Autodesk Fusion 360 part; units mm, degrees
(part 5 of 8)
  spline S142 degree 5 poles (498.6725, -294.9889) (498.7009, -294.8971) (498.7576, -294.7134) (498.842, -294.4377) (498.9535, -294.0701) (499.0912, -293.6105) (499.227, -293.1507) (499.3612, -292.6907) (499.4936, -292.2306) (499.6242, -291.7704) (499.753, -291.31) (499.88, -290.8494) (500.0052, -290.3888) (500.1286, -289.928) (500.2501, -289.4671) (500.3698, -289.006) (500.4876, -288.5449) (500.6035, -288.0836) (500.7175, -287.6223) (500.8296, -287.1608) (500.9398, -286.6992) (501.048, -286.2376) (501.1543, -285.7758) (501.2586, -285.314) (501.3609, -284.8521) (501.4612, -284.3901) (501.5595, -283.9281) (501.6557, -283.4659) (501.7499, -283.0038) (501.842, -282.5415) (501.9319, -282.0793) (502.0198, -281.617) (502.1054, -281.1546) (502.1889, -280.6922) (502.2703, -280.2298) (502.3493, -279.7674) (502.4262, -279.305) (502.5007, -278.8425) (502.5729, -278.3801) (502.6428, -277.9177) (502.7103, -277.4553) (502.7755, -276.9929) (502.8382, -276.5306) (502.8984, -276.0683) (502.9562, -275.606) (503.0114, -275.1439) (503.0639, -274.6817) (503.1139, -274.2197) (503.1611, -273.7578) (503.2055, -273.2959) (503.2472, -272.8342) (503.2861, -272.3726) (503.3222, -271.9111) (503.3553, -271.4498) (503.3854, -270.9886) (503.4124, -270.5277) (503.436, -270.0669) (503.4562, -269.6064) (503.4729, -269.1461) (503.4861, -268.6861) (503.4957, -268.2264) (503.501, -267.8309) (503.5031, -267.5274) (503.5035, -267.3158) (503.5034, -267.1961) (503.5034, -267.1682) knots -1 -1 -1 -1 -1 -1 -0.98571429 -0.97142857 -0.95714286 -0.94285714 -0.92857143 -0.91428571 -0.9 -0.88571429 -0.87142857 -0.85714286 -0.84285714 -0.82857143 -0.81428571 -0.8 -0.78571429 -0.77142857 -0.75714286 -0.74285714 -0.72857143 -0.71428571 -0.7 -0.68571429 -0.67142857 -0.65714286 -0.64285714 -0.62857143 -0.61428571 -0.6 -0.58571429 -0.57142857 -0.55714286 -0.54285714 -0.52857143 -0.51428571 -0.5 -0.48571429 -0.47142857 -0.45714286 -0.44285714 -0.42857143 -0.41428571 -0.4 -0.38571429 -0.37142857 -0.35714286 -0.34285714 -0.32857143 -0.31428571 -0.3 -0.28571429 -0.27142857 -0.25714286 -0.24285714 -0.22857143 -0.21428571 -0.2 -0.18571429 -0.17142857 -0.15714286 -0.14285714 -0.13851185 -0.13851185 -0.13851185 -0.13851185 -0.13851185 -0.13851185
  spline S143 degree 3 poles (504.8034, -265.6048) (504.6001, -265.6422) (504.406, -265.719) (504.0583, -265.9427) (503.908, -266.0874) (503.6968, -266.3896) (503.6248, -266.5359) (503.5278, -266.8451) (503.5032, -267.0062) (503.5034, -267.1682) knots 0 0 0 0 0.062015 0.062015 0.12403 0.12403 0.172638 0.172638 0.221247 0.221247 0.221247 0.221247
  arc A72 (504.8034, -265.6048) -> (512.8852, -263.9972) centre (452.3696, 19.1166) ccw
  spline S144 degree 3 poles (514.6845, -264.9442) (514.6056, -264.7531) (514.4902, -264.5792) (514.1992, -264.2855) (514.0265, -264.1685) (513.6869, -264.0247) (513.5289, -263.9847) (513.2063, -263.954) (513.0436, -263.9634) (512.8852, -263.9972) knots 0 0 0 0 0.062015 0.062015 0.12403 0.12403 0.172638 0.172638 0.221247 0.221247 0.221247 0.221247
  spline S145 degree 5 poles (514.6845, -264.9442) (514.6951, -264.97) (514.7409, -265.0806) (514.8222, -265.2759) (514.9403, -265.5554) (515.0965, -265.9188) (515.2814, -266.3399) (515.4696, -266.7598) (515.6611, -267.1787) (515.856, -267.5964) (516.0542, -268.013) (516.2555, -268.4286) (516.4598, -268.8432) (516.6669, -269.2567) (516.8768, -269.6693) (517.0894, -270.0808) (517.3047, -270.4915) (517.5225, -270.9011) (517.7429, -271.3098) (517.9658, -271.7176) (518.1912, -272.1244) (518.4191, -272.5303) (518.6493, -272.9353) (518.8819, -273.3393) (519.1168, -273.7425) (519.3539, -274.1447) (519.5932, -274.5461) (519.8347, -274.9465) (520.0784, -275.3461) (520.3243, -275.7448) (520.5722, -276.1427) (520.8222, -276.5396) (521.0743, -276.9357) (521.3284, -277.3309) (521.5845, -277.7253) (521.8426, -278.1188) (522.1026, -278.5115) (522.3645, -278.9033) (522.6284, -279.2942) (522.8941, -279.6843) (523.1617, -280.0736) (523.4312, -280.4621) (523.7025, -280.8496) (523.9756, -281.2364) (524.2505, -281.6223) (524.5272, -282.0074) (524.8056, -282.3917) (525.0858, -282.7751) (525.3677, -283.1577) (525.6513, -283.5395) (525.9366, -283.9205) (526.2236, -284.3006) (526.5122, -284.68) (526.8025, -285.0585) (527.0945, -285.4361) (527.3881, -285.813) (527.6833, -286.1891) (527.9801, -286.5643) (528.2784, -286.9387) (528.5784, -287.3123) (528.8799, -287.6851) (529.183, -288.0571) (529.4267, -288.3541) (529.6101, -288.5764) (529.7328, -288.7245) (529.7942, -288.7985) knots 0.13851185 0.13851185 0.13851185 0.13851185 0.13851185 0.13851185 0.14285714 0.15714286 0.17142857 0.18571429 0.2 0.21428571 0.22857143 0.24285714 0.25714286 0.27142857 0.28571429 0.3 0.31428571 0.32857143 0.34285714 0.35714286 0.37142857 0.38571429 0.4 0.41428571 0.42857143 0.44285714 0.45714286 0.47142857 0.48571429 0.5 0.51428571 0.52857143 0.54285714 0.55714286 0.57142857 0.58571429 0.6 0.61428571 0.62857143 0.64285714 0.65714286 0.67142857 0.68571429 0.7 0.71428571 0.72857143 0.74285714 0.75714286 0.77142857 0.78571429 0.8 0.81428571 0.82857143 0.84285714 0.85714286 0.87142857 0.88571429 0.9 0.91428571 0.92857143 0.94285714 0.95714286 0.97142857 0.98571429 1 1 1 1 1 1
  arc A73 (529.7942, -288.7985) -> (539.2754, -286.258) centre (452.3696, 19.1166) ccw
  spline S146 degree 5 poles (539.2754, -286.258) (539.2916, -286.1632) (539.3237, -285.9737) (539.3715, -285.6894) (539.434, -285.3104) (539.5105, -284.8367) (539.5852, -284.3631) (539.6582, -283.8895) (539.7294, -283.4161) (539.7988, -282.9427) (539.8664, -282.4695) (539.9322, -281.9963) (539.9962, -281.5232) (540.0584, -281.0503) (540.1187, -280.5774) (540.1772, -280.1047) (540.2338, -279.6322) (540.2885, -279.1597) (540.3413, -278.6874) (540.3923, -278.2153) (540.4412, -277.7433) (540.4883, -277.2714) (540.5334, -276.7998) (540.5765, -276.3283) (540.6177, -275.8569) (540.6568, -275.3858) (540.694, -274.9149) (540.729, -274.4442) (540.7621, -273.9737) (540.793, -273.5034) (540.8219, -273.0333) (540.8486, -272.5635) (540.8732, -272.0939) (540.8956, -271.6246) (540.9159, -271.1555) (540.9339, -270.6867) (540.9497, -270.2182) (540.9633, -269.75) (540.9745, -269.2821) (540.9835, -268.8146) (540.9901, -268.3473) (540.9943, -267.8804) (540.9961, -267.4138) (540.9955, -266.9476) (540.9924, -266.4818) (540.9868, -266.0163) (540.9786, -265.5513) (540.9678, -265.0867) (540.9543, -264.6226) (540.9381, -264.1589) (540.9192, -263.6957) (540.8975, -263.2329) (540.873, -262.7707) (540.8457, -262.309) (540.8153, -261.8478) (540.7819, -261.3873) (540.7452, -260.9274) (540.7051, -260.4682) (540.6615, -260.0097) (540.6146, -259.5519) (540.5641, -259.0948) (540.5177, -258.702) (540.4802, -258.4008) (540.453, -258.191) (540.4373, -258.0724) (540.4336, -258.0447) knots -1 -1 -1 -1 -1 -1 -0.98571429 -0.97142857 -0.95714286 -0.94285714 -0.92857143 -0.91428571 -0.9 -0.88571429 -0.87142857 -0.85714286 -0.84285714 -0.82857143 -0.81428571 -0.8 -0.78571429 -0.77142857 -0.75714286 -0.74285714 -0.72857143 -0.71428571 -0.7 -0.68571429 -0.67142857 -0.65714286 -0.64285714 -0.62857143 -0.61428571 -0.6 -0.58571429 -0.57142857 -0.55714286 -0.54285714 -0.52857143 -0.51428571 -0.5 -0.48571429 -0.47142857 -0.45714286 -0.44285714 -0.42857143 -0.41428571 -0.4 -0.38571429 -0.37142857 -0.35714286 -0.34285714 -0.32857143 -0.31428571 -0.3 -0.28571429 -0.27142857 -0.25714286 -0.24285714 -0.22857143 -0.21428571 -0.2 -0.18571429 -0.17142857 -0.15714286 -0.14285714 -0.13851185 -0.13851185 -0.13851185 -0.13851185 -0.13851185 -0.13851185
  spline S147 degree 3 poles (541.5184, -256.325) (541.3217, -256.3886) (541.1394, -256.4901) (540.8238, -256.7572) (540.6936, -256.9203) (540.5237, -257.2476) (540.4715, -257.4019) (540.4156, -257.7211) (540.4122, -257.8841) (540.4336, -258.0447) knots 0 0 0 0 0.062015 0.062015 0.12403 0.12403 0.172638 0.172638 0.221247 0.221247 0.221247 0.221247
  arc A74 (541.5184, -256.325) -> (549.3212, -253.6763) centre (452.3696, 19.1166) ccw
  spline S148 degree 3 poles (551.2287, -254.3803) (551.1256, -254.2011) (550.9885, -254.0438) (550.6617, -253.7906) (550.4751, -253.6971) (550.1197, -253.5988) (549.9578, -253.5798) (549.634, -253.5915) (549.4739, -253.622) (549.3212, -253.6763) knots 0 0 0 0 0.062015 0.062015 0.12403 0.12403 0.172638 0.172638 0.221247 0.221247 0.221247 0.221247
  spline S149 degree 5 poles (551.2287, -254.3803) (551.2427, -254.4044) (551.3024, -254.5082) (551.4086, -254.6911) (551.5621, -254.9529) (551.7645, -255.2928) (552.0027, -255.6861) (552.2441, -256.0779) (552.4887, -256.4682) (552.7364, -256.8569) (552.9873, -257.2441) (553.2411, -257.6298) (553.4978, -258.0142) (553.7571, -258.3971) (554.0191, -258.7788) (554.2836, -259.1591) (554.5506, -259.5381) (554.82, -259.9158) (555.0918, -260.2923) (555.3661, -260.6674) (555.6427, -261.0413) (555.9216, -261.414) (556.2027, -261.7855) (556.486, -262.1557) (556.7715, -262.5247) (557.0591, -262.8926) (557.3488, -263.2593) (557.6405, -263.6248) (557.9343, -263.9892) (558.23, -264.3524) (558.5278, -264.7144) (558.8275, -265.0754) (559.1291, -265.4352) (559.4326, -265.7938) (559.738, -266.1514) (560.0452, -266.5079) (560.3543, -266.8632) (560.6651, -267.2175) (560.9777, -267.5707) (561.2921, -267.9228) (561.6083, -268.2738) (561.9261, -268.6237) (562.2457, -268.9726) (562.5669, -269.3204) (562.8898, -269.6671) (563.2144, -270.0128) (563.5406, -270.3574) (563.8684, -270.701) (564.1979, -271.0436) (564.5289, -271.3851) (564.8615, -271.7255) (565.1956, -272.065) (565.5313, -272.4034) (565.8686, -272.7407) (566.2073, -273.0771) (566.5476, -273.4124) (566.8893, -273.7467) (567.2326, -274.08) (567.5773, -274.4123) (567.9234, -274.7435) (568.271, -275.0738) (568.62, -275.403) (568.9004, -275.6656) (569.1113, -275.8621) (569.2522, -275.9929) (569.3228, -276.0583) knots 0.13851185 0.13851185 0.13851185 0.13851185 0.13851185 0.13851185 0.14285714 0.15714286 0.17142857 0.18571429 0.2 0.21428571 0.22857143 0.24285714 0.25714286 0.27142857 0.28571429 0.3 0.31428571 0.32857143 0.34285714 0.35714286 0.37142857 0.38571429 0.4 0.41428571 0.42857143 0.44285714 0.45714286 0.47142857 0.48571429 0.5 0.51428571 0.52857143 0.54285714 0.55714286 0.57142857 0.58571429 0.6 0.61428571 0.62857143 0.64285714 0.65714286 0.67142857 0.68571429 0.7 0.71428571 0.72857143 0.74285714 0.75714286 0.77142857 0.78571429 0.8 0.81428571 0.82857143 0.84285714 0.85714286 0.87142857 0.88571429 0.9 0.91428571 0.92857143 0.94285714 0.95714286 0.97142857 0.98571429 1 1 1 1 1 1
  arc A75 (569.3228, -276.0583) -> (578.3913, -272.302) centre (452.3696, 19.1166) ccw
  spline S150 degree 5 poles (578.3913, -272.302) (578.395, -272.2059) (578.4021, -272.0138) (578.4123, -271.7257) (578.4249, -271.3417) (578.4389, -270.8621) (578.4511, -270.3828) (578.4617, -269.9038) (578.4704, -269.4251) (578.4775, -268.9468) (578.4827, -268.4687) (578.4862, -267.991) (578.4879, -267.5136) (578.4878, -267.0366) (578.4859, -266.5599) (578.4822, -266.0837) (578.4766, -265.6077) (578.4692, -265.1322) (578.4599, -264.657) (578.4488, -264.1823) (578.4358, -263.7079) (578.4208, -263.234) (578.404, -262.7605) (578.3852, -262.2874) (578.3645, -261.8147) (578.3418, -261.3425) (578.3171, -260.8708) (578.2905, -260.3995) (578.2618, -259.9287) (578.2311, -259.4584) (578.1984, -258.9886) (578.1635, -258.5193) (578.1266, -258.0505) (578.0876, -257.5823) (578.0465, -257.1146) (578.0032, -256.6475) (577.9577, -256.1809) (577.91, -255.7149) (577.8601, -255.2496) (577.8079, -254.7848) (577.7535, -254.3207) (577.6967, -253.8572) (577.6376, -253.3944) (577.5762, -252.9323) (577.5123, -252.4708) (577.446, -252.0101) (577.3772, -251.5501) (577.3058, -251.0909) (577.2319, -250.6325) (577.1553, -250.1749) (577.0761, -249.7181) (576.9942, -249.2622) (576.9096, -248.8071) (576.8222, -248.3529) (576.7319, -247.8997) (576.6386, -247.4474) (576.5422, -246.9962) (576.4425, -246.5462) (576.3395, -246.0973) (576.2331, -245.6495) (576.1235, -245.203) (576.0262, -244.8196) (575.9497, -244.5259) (575.8953, -244.3214) (575.8643, -244.2058) (575.857, -244.1789) knots -1 -1 -1 -1 -1 -1 -0.98571429 -0.97142857 -0.95714286 -0.94285714 -0.92857143 -0.91428571 -0.9 -0.88571429 -0.87142857 -0.85714286 -0.84285714 -0.82857143 -0.81428571 -0.8 -0.78571429 -0.77142857 -0.75714286 -0.74285714 -0.72857143 -0.71428571 -0.7 -0.68571429 -0.67142857 -0.65714286 -0.64285714 -0.62857143 -0.61428571 -0.6 -0.58571429 -0.57142857 -0.55714286 -0.54285714 -0.52857143 -0.51428571 -0.5 -0.48571429 -0.47142857 -0.45714286 -0.44285714 -0.42857143 -0.41428571 -0.4 -0.38571429 -0.37142857 -0.35714286 -0.34285714 -0.32857143 -0.31428571 -0.3 -0.28571429 -0.27142857 -0.25714286 -0.24285714 -0.22857143 -0.21428571 -0.2 -0.18571429 -0.17142857 -0.15714286 -0.14285714 -0.13851185 -0.13851185 -0.13851185 -0.13851185 -0.13851185 -0.13851185
  spline S151 degree 3 poles (576.7081, -242.3323) (576.5214, -242.4211) (576.3538, -242.5455) (576.0758, -242.8515) (575.9681, -243.0302) (575.8423, -243.3768) (575.8107, -243.5367) (575.7969, -243.8604) (575.8149, -244.0224) (575.857, -244.1789) knots 0 0 0 0 0.062015 0.062015 0.12403 0.12403 0.172638 0.172638 0.221247 0.221247 0.221247 0.221247
  arc A76 (576.7081, -242.3323) -> (584.0984, -238.6878) centre (452.3696, 19.1166) ccw
  spline S152 degree 3 poles (586.0815, -239.1367) (585.9559, -238.9726) (585.7994, -238.8345) (585.4423, -238.6261) (585.2451, -238.5578) (584.8799, -238.5068) (584.717, -238.5091) (584.3974, -238.5628) (584.2427, -238.6141) (584.0984, -238.6878) knots 0 0 0 0 0.062015 0.062015 0.12403 0.12403 0.172638 0.172638 0.221247 0.221247 0.221247 0.221247
  spline S153 degree 5 poles (586.0815, -239.1367) (586.0984, -239.1589) (586.1713, -239.2539) (586.3004, -239.4215) (586.4868, -239.661) (586.7317, -239.9716) (587.0193, -240.3304) (587.3097, -240.6873) (587.6032, -241.0423) (587.8996, -241.3954) (588.1988, -241.7465) (588.5008, -242.0959) (588.8054, -242.4434) (589.1125, -242.7892) (589.4221, -243.1334) (589.734, -243.4759) (590.0481, -243.8169) (590.3646, -244.1562) (590.6832, -244.4939) (591.0041, -244.8301) (591.3271, -245.1647) (591.6523, -245.4978) (591.9795, -245.8294) (592.3087, -246.1595) (592.6399, -246.4881) (592.973, -246.8153) (593.3081, -247.141) (593.6451, -247.4653) (593.9839, -247.7882) (594.3245, -248.1097) (594.667, -248.4298) (595.0112, -248.7485) (595.3572, -249.0659) (595.7049, -249.3819) (596.0544, -249.6965) (596.4055, -250.0098) (596.7583, -250.3218) (597.1127, -250.6325) (597.4688, -250.9418) (597.8264, -251.2498) (598.1857, -251.5566) (598.5465, -251.8621) (598.9088, -252.1662) (599.2727, -252.4691) (599.6382, -252.7707) (600.0051, -253.0711) (600.3735, -253.3702) (600.7433, -253.6681) (601.1147, -253.9647) (601.4874, -254.2601) (601.8616, -254.5542) (602.2372, -254.8471) (602.6142, -255.1388) (602.9926, -255.4293) (603.3723, -255.7185) (603.7535, -256.0066) (604.1359, -256.2934) (604.5197, -256.579) (604.9048, -256.8635) (605.2913, -257.1467) (605.679, -257.4288) (606.068, -257.7097) (606.3803, -257.9334) (606.615, -258.1007) (606.7718, -258.212) (606.8503, -258.2676) knots 0.13851185 0.13851185 0.13851185 0.13851185 0.13851185 0.13851185 0.14285714 0.15714286 0.17142857 0.18571429 0.2 0.21428571 0.22857143 0.24285714 0.25714286 0.27142857 0.28571429 0.3 0.31428571 0.32857143 0.34285714 0.35714286 0.37142857 0.38571429 0.4 0.41428571 0.42857143 0.44285714 0.45714286 0.47142857 0.48571429 0.5 0.51428571 0.52857143 0.54285714 0.55714286 0.57142857 0.58571429 0.6 0.61428571 0.62857143 0.64285714 0.65714286 0.67142857 0.68571429 0.7 0.71428571 0.72857143 0.74285714 0.75714286 0.77142857 0.78571429 0.8 0.81428571 0.82857143 0.84285714 0.85714286 0.87142857 0.88571429 0.9 0.91428571 0.92857143 0.94285714 0.95714286 0.97142857 0.98571429 1 1 1 1 1 1
  arc A77 (606.8503, -258.2676) -> (615.3509, -253.3597) centre (452.3696, 19.1166) ccw
  spline S154 degree 5 poles (615.3509, -253.3597) (615.342, -253.264) (615.324, -253.0726) (615.2965, -252.7856) (615.2589, -252.4033) (615.2101, -251.926) (615.1597, -251.4492) (615.1077, -250.9729) (615.0539, -250.4971) (614.9984, -250.0219) (614.9412, -249.5473) (614.8823, -249.0732) (614.8217, -248.5997) (614.7594, -248.1268) (614.6953, -247.6545) (614.6294, -247.1827) (614.5618, -246.7116) (614.4923, -246.2411) (614.4211, -245.7712) (614.3481, -245.302) (614.2733, -244.8334) (614.1966, -244.3654) (614.1181, -243.8982) (614.0377, -243.4316) (613.9555, -242.9657) (613.8713, -242.5005) (613.7853, -242.036) (613.6974, -241.5722) (613.6075, -241.1092) (613.5157, -240.6469) (613.4219, -240.1854) (613.3261, -239.7247) (613.2283, -239.2647) (613.1285, -238.8056) (613.0267, -238.3473) (612.9228, -237.8898) (612.8168, -237.4332) (612.7087, -236.9774) (612.5985, -236.5225) (612.4861, -236.0686) (612.3715, -235.6155) (612.2548, -235.1634) (612.1358, -234.7123) (612.0145, -234.2621) (611.891, -233.813) (611.7651, -233.3648) (611.6368, -232.9178) (611.5061, -232.4718) (611.373, -232.027) (611.2373, -231.5833) (611.0991, -231.1407) (610.9584, -230.6994) (610.8152, -230.2592) (610.6692, -229.8203) (610.5206, -229.3828) (610.369, -228.9466) (610.2145, -228.5118) (610.057, -228.0786) (609.8963, -227.647) (609.7324, -227.217) (609.5654, -226.7886) (609.4189, -226.4211) (609.3047, -226.14) (609.2241, -225.9443) (609.1782, -225.8338) (609.1675, -225.808) knots -1 -1 -1 -1 -1 -1 -0.98571429 -0.97142857 -0.95714286 -0.94285714 -0.92857143 -0.91428571 -0.9 -0.88571429 -0.87142857 -0.85714286 -0.84285714 -0.82857143 -0.81428571 -0.8 -0.78571429 -0.77142857 -0.75714286 -0.74285714 -0.72857143 -0.71428571 -0.7 -0.68571429 -0.67142857 -0.65714286 -0.64285714 -0.62857143 -0.61428571 -0.6 -0.58571429 -0.57142857 -0.55714286 -0.54285714 -0.52857143 -0.51428571 -0.5 -0.48571429 -0.47142857 -0.45714286 -0.44285714 -0.42857143 -0.41428571 -0.4 -0.38571429 -0.37142857 -0.35714286 -0.34285714 -0.32857143 -0.31428571 -0.3 -0.28571429 -0.27142857 -0.25714286 -0.24285714 -0.22857143 -0.21428571 -0.2 -0.18571429 -0.17142857 -0.15714286 -0.14285714 -0.13851185 -0.13851185 -0.13851185 -0.13851185 -0.13851185 -0.13851185
  spline S155 degree 3 poles (609.7703, -223.8661) (609.5968, -223.9785) (609.4469, -224.1237) (609.2112, -224.4634) (609.1277, -224.6546) (609.0482, -225.0147) (609.0377, -225.1773) (609.0664, -225.5001) (609.1053, -225.6584) (609.1675, -225.808) knots 0 0 0 0 0.062015 0.062015 0.12403 0.12403 0.172638 0.172638 0.221247 0.221247 0.221247 0.221247
  arc A78 (609.7703, -223.8661) -> (616.6217, -219.2882) centre (452.3696, 19.1166) ccw
  spline S156 degree 3 poles (618.6464, -219.4744) (618.5004, -219.3281) (618.3272, -219.2116) (617.946, -219.0516) (617.7416, -219.0096) (617.3729, -219.0067) (617.2116, -219.0302) (616.9018, -219.1253) (616.7551, -219.1962) (616.6217, -219.2882) knots 0 0 0 0 0.062015 0.062015 0.12403 0.12403 0.172638 0.172638 0.221247 0.221247 0.221247 0.221247
  spline S157 degree 5 poles (618.6464, -219.4744) (618.6661, -219.4942) (618.7507, -219.5789) (618.9006, -219.7282) (619.1166, -219.9413) (619.4, -220.2172) (619.732, -220.5355) (620.0665, -220.8515) (620.4038, -221.1651) (620.7437, -221.4765) (621.0862, -221.7856) (621.4312, -222.0925) (621.7786, -222.3973) (622.1283, -222.7001) (622.4801, -223.0009) (622.834, -223.2998) (623.19, -223.5968) (623.548, -223.8919) (623.908, -224.1851) (624.27, -224.4766) (624.6339, -224.7661) (624.9998, -225.0539) (625.3675, -225.34) (625.737, -225.6243) (626.1082, -225.9068) (626.4812, -226.1877) (626.8559, -226.4669) (627.2323, -226.7445) (627.6104, -227.0204) (627.9901, -227.2947) (628.3714, -227.5674) (628.7543, -227.8384) (629.1388, -228.1079) (629.5248, -228.3758) (629.9123, -228.6421) (630.3013, -228.9069) (630.6918, -229.1702) (631.0837, -229.4319) (631.4771, -229.6922) (631.8719, -229.9509) (632.2681, -230.2081) (632.6657, -230.4639) (633.0647, -230.7181) (633.465, -230.971) (633.8667, -231.2223) (634.2697, -231.4722) (634.6739, -231.7207) (635.0795, -231.9677) (635.4864, -232.2133) (635.8945, -232.4575) (636.3039, -232.7003) (636.7145, -232.9417) (637.1263, -233.1817) (637.5394, -233.4202) (637.9537, -233.6575) (638.3691, -233.8933) (638.7858, -234.1277) (639.2036, -234.3608) (639.6225, -234.5926) (640.0426, -234.823) (640.4638, -235.052) (640.8862, -235.2797) (641.225, -235.4608) (641.4796, -235.596) (641.6495, -235.6859) (641.7345, -235.7307) knots 0.13851185 0.13851185 0.13851185 0.13851185 0.13851185 0.13851185 0.14285714 0.15714286 0.17142857 0.18571429 0.2 0.21428571 0.22857143 0.24285714 0.25714286 0.27142857 0.28571429 0.3 0.31428571 0.32857143 0.34285714 0.35714286 0.37142857 0.38571429 0.4 0.41428571 0.42857143 0.44285714 0.45714286 0.47142857 0.48571429 0.5 0.51428571 0.52857143 0.54285714 0.55714286 0.57142857 0.58571429 0.6 0.61428571 0.62857143 0.64285714 0.65714286 0.67142857 0.68571429 0.7 0.71428571 0.72857143 0.74285714 0.75714286 0.77142857 0.78571429 0.8 0.81428571 0.82857143 0.84285714 0.85714286 0.87142857 0.88571429 0.9 0.91428571 0.92857143 0.94285714 0.95714286 0.97142857 0.98571429 1 1 1 1 1 1
  arc A79 (641.7345, -235.7307) -> (649.5219, -229.7553) centre (452.3696, 19.1166) ccw
  spline S158 degree 5 poles (649.5219, -229.7553) (649.5006, -229.6615) (649.4577, -229.4741) (649.393, -229.1932) (649.3058, -228.8191) (649.1952, -228.3522) (649.083, -227.8861) (648.9692, -227.4206) (648.8538, -226.956) (648.7367, -226.4921) (648.6181, -226.029) (648.4978, -225.5666) (648.3759, -225.1051) (648.2524, -224.6444) (648.1272, -224.1844) (648.0003, -223.7253) (647.8717, -223.2671) (647.7415, -222.8097) (647.6095, -222.3531) (647.4759, -221.8974) (647.3405, -221.4426) (647.2034, -220.9886) (647.0646, -220.5356) (646.924, -220.0835) (646.7817, -219.6323) (646.6376, -219.1821) (646.4916, -218.7328) (646.3439, -218.2845) (646.1944, -217.8372) (646.043, -217.3908) (645.8898, -216.9455) (645.7347, -216.5012) (645.5777, -216.058) (645.4188, -215.6158) (645.258, -215.1747) (645.0953, -214.7347) (644.9306, -214.2958) (644.764, -213.858) (644.5953, -213.4214) (644.4246, -212.986) (644.2519, -212.5518) (644.0771, -212.1188) (643.9003, -211.6871) (643.7213, -211.2566) (643.5402, -210.8274) (643.3569, -210.3995) (643.1713, -209.973) (642.9836, -209.5479) (642.7935, -209.1243) (642.6011, -208.7021) (642.4063, -208.2814) (642.2092, -207.8622) (642.0097, -207.4445) (641.8077, -207.0284) (641.6032, -206.614) (641.3961, -206.2013) (641.1861, -205.7904) (640.9734, -205.3815) (640.7577, -204.9746) (640.5391, -204.5696) (640.3176, -204.1666) (640.1244, -203.8215) (639.9745, -203.5576) (639.8691, -203.3742) (639.8092, -203.2706) (639.7952, -203.2464) knots -1 -1 -1 -1 -1 -1 -0.98571429 -0.97142857 -0.95714286 -0.94285714 -0.92857143 -0.91428571 -0.9 -0.88571429 -0.87142857 -0.85714286 -0.84285714 -0.82857143 -0.81428571 -0.8 -0.78571429 -0.77142857 -0.75714286 -0.74285714 -0.72857143 -0.71428571 -0.7 -0.68571429 -0.67142857 -0.65714286 -0.64285714 -0.62857143 -0.61428571 -0.6 -0.58571429 -0.57142857 -0.55714286 -0.54285714 -0.52857143 -0.51428571 -0.5 -0.48571429 -0.47142857 -0.45714286 -0.44285714 -0.42857143 -0.41428571 -0.4 -0.38571429 -0.37142857 -0.35714286 -0.34285714 -0.32857143 -0.31428571 -0.3 -0.28571429 -0.27142857 -0.25714286 -0.24285714 -0.22857143 -0.21428571 -0.2 -0.18571429 -0.17142857 -0.15714286 -0.14285714 -0.13851185 -0.13851185 -0.13851185 -0.13851185 -0.13851185 -0.13851185
  spline S159 degree 3 poles (640.1393, -201.2425) (639.9819, -201.3765) (639.8523, -201.54) (639.663, -201.9076) (639.6051, -202.1081) (639.5733, -202.4755) (639.5842, -202.6381) (639.6547, -202.9544) (639.714, -203.1062) (639.7952, -203.2464) knots 0 0 0 0 0.062015 0.062015 0.12403 0.12403 0.172638 0.172638 0.221247 0.221247 0.221247 0.221247
  arc A80 (640.1393, -201.2425) -> (646.3345, -195.8094) centre (452.3696, 19.1166) ccw
  spline S160 degree 3 poles (648.3662, -195.7298) (648.2024, -195.6037) (648.0155, -195.5108) (647.6167, -195.402) (647.4085, -195.387) (647.0426, -195.4323) (646.8858, -195.4766) (646.591, -195.6113) (646.4548, -195.7008) (646.3345, -195.8094) knots 0 0 0 0 0.062015 0.062015 0.12403 0.12403 0.172638 0.172638 0.221247 0.221247 0.221247 0.221247
  spline S161 degree 5 poles (648.3662, -195.7298) (648.3884, -195.7468) (648.4833, -195.8197) (648.6514, -195.9482) (648.8934, -196.1313) (649.2104, -196.3678) (649.581, -196.6401) (649.954, -196.9096) (650.3293, -197.1766) (650.7069, -197.4409) (651.0869, -197.7027) (651.469, -197.9619) (651.8532, -198.2188) (652.2394, -198.4733) (652.6274, -198.7256) (653.0173, -198.9758) (653.409, -199.2238) (653.8025, -199.4696) (654.1977, -199.7134) (654.5946, -199.9551) (654.9933, -200.1947) (655.3935, -200.4323) (655.7954, -200.6678) (656.1989, -200.9015) (656.6038, -201.1332) (657.0103, -201.363) (657.4183, -201.5909) (657.8277, -201.817) (658.2385, -202.0412) (658.6508, -202.2635) (659.0644, -202.4841) (659.4794, -202.7029) (659.8958, -202.9198) (660.3134, -203.1351) (660.7324, -203.3486) (661.1526, -203.5603) (661.5741, -203.7704) (661.9969, -203.9787) (662.4209, -204.1853) (662.8461, -204.3903) (663.2725, -204.5936) (663.7001, -204.7953) (664.1288, -204.9953) (664.5587, -205.1937) (664.9897, -205.3905) (665.4219, -205.5857) (665.8551, -205.7792) (666.2895, -205.9712) (666.7249, -206.1616) (667.1614, -206.3504) (667.599, -206.5377) (668.0376, -206.7234) (668.4773, -206.9076) (668.9179, -207.0902) (669.3596, -207.2713) (669.8023, -207.4509) (670.246, -207.629) (670.6906, -207.8056) (671.1362, -207.9807) (671.5828, -208.1542) (672.0303, -208.3263) (672.4788, -208.4969) (672.8383, -208.6323) (673.1084, -208.7331) (673.2886, -208.8) (673.3787, -208.8334) knots 0.13851185 0.13851185 0.13851185 0.13851185 0.13851185 0.13851185 0.14285714 0.15714286 0.17142857 0.18571429 0.2 0.21428571 0.22857143 0.24285714 0.25714286 0.27142857 0.28571429 0.3 0.31428571 0.32857143 0.34285714 0.35714286 0.37142857 0.38571429 0.4 0.41428571 0.42857143 0.44285714 0.45714286 0.47142857 0.48571429 0.5 0.51428571 0.52857143 0.54285714 0.55714286 0.57142857 0.58571429 0.6 0.61428571 0.62857143 0.64285714 0.65714286 0.67142857 0.68571429 0.7 0.71428571 0.72857143 0.74285714 0.75714286 0.77142857 0.78571429 0.8 0.81428571 0.82857143 0.84285714 0.85714286 0.87142857 0.88571429 0.9 0.91428571 0.92857143 0.94285714 0.95714286 0.97142857 0.98571429 1 1 1 1 1 1
  arc A81 (673.3787, -208.8334) -> (680.3195, -201.8926) centre (452.3696, 19.1166) ccw
  spline S162 degree 5 poles (680.3195, -201.8926) (680.2861, -201.8024) (680.2192, -201.6222) (680.1184, -201.3522) (679.9831, -200.9926) (679.8125, -200.5442) (679.6404, -200.0967) (679.4668, -199.6501) (679.2917, -199.2045) (679.1151, -198.7598) (678.9371, -198.3162) (678.7575, -197.8735) (678.5764, -197.4318) (678.3937, -196.9911) (678.2096, -196.5515) (678.0239, -196.1129) (677.8366, -195.6753) (677.6478, -195.2388) (677.4573, -194.8033) (677.2654, -194.369) (677.0718, -193.9357) (676.8766, -193.5036) (676.6799, -193.0726) (676.4815, -192.6427) (676.2814, -192.2139) (676.0798, -191.7863) (675.8765, -191.3599) (675.6715, -190.9347) (675.4648, -190.5108) (675.2565, -190.088) (675.0464, -189.6665) (674.8347, -189.2463) (674.6212, -188.8273) (674.406, -188.4096) (674.189, -187.9933) (673.9702, -187.5783) (673.7497, -187.1646) (673.5273, -186.7524) (673.3031, -186.3415) (673.077, -185.9321) (672.8491, -185.5242) (672.6193, -185.1177) (672.3876, -184.7127) (672.154, -184.3093) (671.9184, -183.9074) (671.6808, -183.5071) (671.4412, -183.1085) (671.1995, -182.7116) (670.9558, -182.3164) (670.7099, -181.9229) (670.4619, -181.5312) (670.2118, -181.1413) (669.9595, -180.7532) (669.7049, -180.367) (669.448, -179.9829) (669.1888, -179.6007) (668.927, -179.2208) (668.6627, -178.8431) (668.3958, -178.4678) (668.1262, -178.0949) (667.854, -177.7243) (667.6174, -177.4073) (667.4343, -177.1652) (667.3059, -176.9971) (667.2329, -176.9022) (667.2159, -176.8801) knots -1 -1 -1 -1 -1 -1 -0.98571429 -0.97142857 -0.95714286 -0.94285714 -0.92857143 -0.91428571 -0.9 -0.88571429 -0.87142857 -0.85714286 -0.84285714 -0.82857143 -0.81428571 -0.8 -0.78571429 -0.77142857 -0.75714286 -0.74285714 -0.72857143 -0.71428571 -0.7 -0.68571429 -0.67142857 -0.65714286 -0.64285714 -0.62857143 -0.61428571 -0.6 -0.58571429 -0.57142857 -0.55714286 -0.54285714 -0.52857143 -0.51428571 -0.5 -0.48571429 -0.47142857 -0.45714286 -0.44285714 -0.42857143 -0.41428571 -0.4 -0.38571429 -0.37142857 -0.35714286 -0.34285714 -0.32857143 -0.31428571 -0.3 -0.28571429 -0.27142857 -0.25714286 -0.24285714 -0.22857143 -0.21428571 -0.2 -0.18571429 -0.17142857 -0.15714286 -0.14285714 -0.13851185 -0.13851185 -0.13851185 -0.13851185 -0.13851185 -0.13851185
  spline S163 degree 3 poles (667.2955, -174.8484) (667.157, -175.0018) (667.0498, -175.1809) (666.9101, -175.57) (666.8789, -175.7763) (666.8954, -176.1447) (666.9273, -176.3045) (667.0385, -176.6089) (667.1171, -176.7517) (667.2159, -176.8801) knots 0 0 0 0 0.062015 0.062015 0.12403 0.12403 0.172638 0.172638 0.221247 0.221247 0.221247 0.221247
  arc A82 (667.2955, -174.8484) -> (672.7286, -168.6531) centre (452.3696, 19.1166) ccw
  spline S164 degree 3 poles (674.7325, -168.309) (674.5537, -168.2054) (674.3563, -168.1378) (673.9466, -168.0819) (673.7383, -168.0942) (673.3814, -168.1868) (673.2317, -168.2513) (672.957, -168.4233) (672.8337, -168.5298) (672.7286, -168.6531) knots 0 0 0 0 0.062015 0.062015 0.12403 0.12403 0.172638 0.172638 0.221247 0.221247 0.221247 0.221247
  spline S165 degree 5 poles (674.7325, -168.309) (674.7567, -168.323) (674.8603, -168.3829) (675.0437, -168.4883) (675.3076, -168.6383) (675.6528, -168.8315) (676.0557, -169.053) (676.4607, -169.2716) (676.8676, -169.4872) (677.2766, -169.7) (677.6874, -169.9099) (678.1001, -170.1171) (678.5145, -170.3216) (678.9306, -170.5236) (679.3483, -170.7231) (679.7675, -170.9202) (680.1882, -171.1149) (680.6104, -171.3073) (681.0341, -171.4974) (681.4592, -171.6852) (681.8857, -171.8707) (682.3135, -172.054) (682.7427, -172.2352) (683.1732, -172.4141) (683.605, -172.591) (684.0379, -172.7658) (684.4722, -172.9385) (684.9076, -173.1092) (685.3442, -173.2778) (685.7819, -173.4445) (686.2208, -173.6092) (686.6608, -173.7719) (687.1019, -173.9327) (687.5441, -174.0916) (687.9873, -174.2485) (688.4316, -174.4036) (688.877, -174.5568) (689.3233, -174.7082) (689.7706, -174.8578) (690.2189, -175.0055) (690.6682, -175.1514) (691.1185, -175.2955) (691.5696, -175.4379) (692.0218, -175.5785) (692.4748, -175.7173) (692.9287, -175.8544) (693.3835, -175.9898) (693.8392, -176.1234) (694.2958, -176.2553) (694.7532, -176.3856) (695.2115, -176.5141) (695.6706, -176.641) (696.1305, -176.7662) (696.5912, -176.8898) (697.0528, -177.0117) (697.5151, -177.132) (697.9782, -177.2506) (698.4421, -177.3676) (698.9068, -177.483) (699.3722, -177.5968) (699.8383, -177.709) (700.3052, -177.8197) (700.6793, -177.9069) (700.9603, -177.9716) (701.1477, -178.0144) (701.2414, -178.0357) knots 0.13851185 0.13851185 0.13851185 0.13851185 0.13851185 0.13851185 0.14285714 0.15714286 0.17142857 0.18571429 0.2 0.21428571 0.22857143 0.24285714 0.25714286 0.27142857 0.28571429 0.3 0.31428571 0.32857143 0.34285714 0.35714286 0.37142857 0.38571429 0.4 0.41428571 0.42857143 0.44285714 0.45714286 0.47142857 0.48571429 0.5 0.51428571 0.52857143 0.54285714 0.55714286 0.57142857 0.58571429 0.6 0.61428571 0.62857143 0.64285714 0.65714286 0.67142857 0.68571429 0.7 0.71428571 0.72857143 0.74285714 0.75714286 0.77142857 0.78571429 0.8 0.81428571 0.82857143 0.84285714 0.85714286 0.87142857 0.88571429 0.9 0.91428571 0.92857143 0.94285714 0.95714286 0.97142857 0.98571429 1 1 1 1 1 1
  arc A83 (701.2414, -178.0357) -> (707.2169, -170.2484) centre (452.3696, 19.1166) ccw
  spline S166 degree 5 poles (707.2169, -170.2484) (707.172, -170.1634) (707.0821, -169.9934) (706.9469, -169.7388) (706.7658, -169.4) (706.5381, -168.9777) (706.3091, -168.5565) (706.0787, -168.1364) (705.847, -167.7174) (705.6139, -167.2996) (705.3794, -166.883) (705.1436, -166.4675) (704.9064, -166.0533) (704.6678, -165.6402) (704.4278, -165.2284) (704.1864, -164.8177) (703.9436, -164.4084) (703.6995, -164.0002) (703.4538, -163.5934) (703.2068, -163.1878) (702.9583, -162.7835) (702.7084, -162.3805) (702.4571, -161.9789) (702.2043, -161.5786) (701.95, -161.1796) (701.6943, -160.782) (701.437, -160.3858) (701.1783, -159.991) (700.9181, -159.5976) (700.6563, -159.2057) (700.3931, -158.8152) (700.1283, -158.4262) (699.8619, -158.0386) (699.594, -157.6526) (699.3246, -157.2682) (699.0535, -156.8853) (698.7808, -156.504) (698.5066, -156.1243) (698.2306, -155.7462) (697.9531, -155.3698) (697.6739, -154.9951) (697.393, -154.6221) (697.1104, -154.2508) (696.8261, -153.8813) (696.5401, -153.5136) (696.2523, -153.1478) (695.9627, -152.7839) (695.6713, -152.4219) (695.378, -152.0618) (695.0829, -151.7038) (694.7859, -151.3478) (694.487, -150.9939) (694.1862, -150.6421) (693.8834, -150.2925) (693.5786, -149.9451) (693.2717, -149.6001) (692.9626, -149.2576) (692.6512, -148.9177) (692.3376, -148.5804) (692.0216, -148.2458) (691.7034, -147.9139) (691.4274, -147.6305) (691.2143, -147.4144) (691.065, -147.2645) (690.9803, -147.18) (690.9606, -147.1602) knots -1 -1 -1 -1 -1 -1 -0.98571429 -0.97142857 -0.95714286 -0.94285714 -0.92857143 -0.91428571 -0.9 -0.88571429 -0.87142857 -0.85714286 -0.84285714 -0.82857143 -0.81428571 -0.8 -0.78571429 -0.77142857 -0.75714286 -0.74285714 -0.72857143 -0.71428571 -0.7 -0.68571429 -0.67142857 -0.65714286 -0.64285714 -0.62857143 -0.61428571 -0.6 -0.58571429 -0.57142857 -0.55714286 -0.54285714 -0.52857143 -0.51428571 -0.5 -0.48571429 -0.47142857 -0.45714286 -0.44285714 -0.42857143 -0.41428571 -0.4 -0.38571429 -0.37142857 -0.35714286 -0.34285714 -0.32857143 -0.31428571 -0.3 -0.28571429 -0.27142857 -0.25714286 -0.24285714 -0.22857143 -0.21428571 -0.2 -0.18571429 -0.17142857 -0.15714286 -0.14285714 -0.13851185 -0.13851185 -0.13851185 -0.13851185 -0.13851185 -0.13851185
  spline S167 degree 3 poles (690.7743, -145.1355) (690.657, -145.3057) (690.5741, -145.4972) (690.4864, -145.9013) (690.4824, -146.1099) (690.5468, -146.473) (690.5993, -146.6273) (690.7493, -146.9145) (690.8458, -147.0458) (690.9606, -147.1602) knots 0 0 0 0 0.062015 0.062015 0.12403 0.12403 0.172638 0.172638 0.221247 0.221247 0.221247 0.221247
  arc A84 (690.7743, -145.1355) -> (695.3523, -138.2841) centre (452.3696, 19.1166) ccw
  spline S168 degree 3 poles (697.2941, -137.6814) (697.1033, -137.602) (696.8987, -137.5607) (696.4853, -137.5588) (696.2804, -137.5982) (695.9386, -137.7366) (695.7986, -137.8201) (695.5487, -138.0264) (695.4403, -138.1481) (695.3523, -138.2841) knots 0 0 0 0 0.062015 0.062015 0.12403 0.12403 0.172638 0.172638 0.221247 0.221247 0.221247 0.221247
  spline S169 degree 5 poles (697.2941, -137.6814) (697.3199, -137.6921) (697.4305, -137.738) (697.6261, -137.8185) (697.9073, -137.9327) (698.2747, -138.0792) (698.7031, -138.2462) (699.1332, -138.4101) (699.5648, -138.5708) (699.998, -138.7284) (700.4327, -138.8829) (700.8689, -139.0344) (701.3065, -139.1831) (701.7454, -139.329) (702.1855, -139.4723) (702.6269, -139.613) (703.0694, -139.7512) (703.5131, -139.8868) (703.958, -140.02) (704.4039, -140.1507) (704.851, -140.2789) (705.2991, -140.4048) (705.7483, -140.5284) (706.1984, -140.6496) (706.6496, -140.7686) (707.1017, -140.8854) (707.5547, -141) (708.0087, -141.1123) (708.4635, -141.2226) (708.9193, -141.3307) (709.3759, -141.4367) (709.8334, -141.5406) (710.2917, -141.6424) (710.7509, -141.7422) (711.2108, -141.84) (711.6715, -141.9357) (712.1331, -142.0295) (712.5953, -142.1214) (713.0584, -142.2112) (713.5221, -142.2992) (713.9866, -142.3852) (714.4518, -142.4693) (714.9177, -142.5516) (715.3843, -142.6319) (715.8516, -142.7105) (716.3195, -142.7871) (716.7881, -142.862) (717.2574, -142.935) (717.7272, -143.0062) (718.1977, -143.0756) (718.6689, -143.1433) (719.1406, -143.2091) (719.6129, -143.2732) (720.0859, -143.3356) (720.5594, -143.3962) (721.0334, -143.4551) (721.5081, -143.5123) (721.9833, -143.5677) (722.459, -143.6215) (722.9353, -143.6736) (723.4121, -143.724) (723.8894, -143.7727) (724.2717, -143.8104) (724.5587, -143.8379) (724.7501, -143.8559) (724.8458, -143.8648) knots 0.13851185 0.13851185 0.13851185 0.13851185 0.13851185 0.13851185 0.14285714 0.15714286 0.17142857 0.18571429 0.2 0.21428571 0.22857143 0.24285714 0.25714286 0.27142857 0.28571429 0.3 0.31428571 0.32857143 0.34285714 0.35714286 0.37142857 0.38571429 0.4 0.41428571 0.42857143 0.44285714 0.45714286 0.47142857 0.48571429 0.5 0.51428571 0.52857143 0.54285714 0.55714286 0.57142857 0.58571429 0.6 0.61428571 0.62857143 0.64285714 0.65714286 0.67142857 0.68571429 0.7 0.71428571 0.72857143 0.74285714 0.75714286 0.77142857 0.78571429 0.8 0.81428571 0.82857143 0.84285714 0.85714286 0.87142857 0.88571429 0.9 0.91428571 0.92857143 0.94285714 0.95714286 0.97142857 0.98571429 1 1 1 1 1 1
  arc A85 (724.8458, -143.8648) -> (729.7537, -135.3641) centre (452.3696, 19.1166) ccw
  spline S170 degree 5 poles (729.7537, -135.3641) (729.6981, -135.2857) (729.5868, -135.1289) (729.4195, -134.8941) (729.1958, -134.5819) (728.9149, -134.1929) (728.6329, -133.8051) (728.3496, -133.4187) (728.0652, -133.0336) (727.7795, -132.6498) (727.4927, -132.2673) (727.2047, -131.8862) (726.9154, -131.5064) (726.6249, -131.1281) (726.3333, -130.7511) (726.0404, -130.3755) (725.7462, -130.0013) (725.4508, -129.6285) (725.1542, -129.2572) (724.8564, -128.8873) (724.5573, -128.5189) (724.2569, -128.152) (723.9553, -127.7866) (723.6524, -127.4227) (723.3482, -127.0603) (723.0427, -126.6995) (722.736, -126.3403) (722.4279, -125.9826) (722.1186, -125.6266) (721.8079, -125.2722) (721.496, -124.9194) (721.1826, -124.5682) (720.868, -124.2188) (720.552, -123.8711) (720.2347, -123.5251) (719.9159, -123.1808) (719.5958, -122.8384) (719.2743, -122.4977) (718.9514, -122.1589) (718.6271, -121.822) (718.3014, -121.4869) (717.9742, -121.1538) (717.6456, -120.8225) (717.3155, -120.4933) (716.9839, -120.1661) (716.6508, -119.841) (716.3162, -119.5179) (715.9801, -119.1971) (715.6423, -118.8784) (715.303, -118.562) (714.9621, -118.2478) (714.6195, -117.9359) (714.2754, -117.6264) (713.9295, -117.3193) (713.582, -117.0147) (713.2327, -116.7127) (712.8815, -116.4134) (712.5285, -116.117) (712.1735, -115.8236) (711.8166, -115.5331) (711.4577, -115.2456) (711.1471, -115.0006) (710.9076, -114.8142) (710.7401, -114.6851) (710.645, -114.6123) (710.6229, -114.5953) knots -1 -1 -1 -1 -1 -1 -0.98571429 -0.97142857 -0.95714286 -0.94285714 -0.92857143 -0.91428571 -0.9 -0.88571429 -0.87142857 -0.85714286 -0.84285714 -0.82857143 -0.81428571 -0.8 -0.78571429 -0.77142857 -0.75714286 -0.74285714 -0.72857143 -0.71428571 -0.7 -0.68571429 -0.67142857 -0.65714286 -0.64285714 -0.62857143 -0.61428571 -0.6 -0.58571429 -0.57142857 -0.55714286 -0.54285714 -0.52857143 -0.51428571 -0.5 -0.48571429 -0.47142857 -0.45714286 -0.44285714 -0.42857143 -0.41428571 -0.4 -0.38571429 -0.37142857 -0.35714286 -0.34285714 -0.32857143 -0.31428571 -0.3 -0.28571429 -0.27142857 -0.25714286 -0.24285714 -0.22857143 -0.21428571 -0.2 -0.18571429 -0.17142857 -0.15714286 -0.14285714 -0.13851185 -0.13851185 -0.13851185 -0.13851185 -0.13851185 -0.13851185
  spline S171 degree 3 poles (710.1739, -112.6123) (710.0799, -112.7963) (710.0227, -112.997) (709.9884, -113.409) (710.0117, -113.6164) (710.1229, -113.968) (710.1952, -114.1141) (710.3813, -114.3793) (710.4942, -114.4969) (710.6229, -114.5953) knots 0 0 0 0 0.062015 0.062015 0.12403 0.12403 0.172638 0.172638 0.221247 0.221247 0.221247 0.221247
  arc A86 (710.1739, -112.6123) -> (713.8184, -105.2219) centre (452.3696, 19.1166) ccw
  spline S172 degree 3 poles (715.665, -104.3709) (715.4654, -104.3171) (715.2572, -104.3028) (714.8471, -104.3549) (714.6491, -104.4207) (714.3283, -104.6026) (714.2004, -104.7036) (713.9796, -104.9408) (713.888, -105.0756) (713.8184, -105.2219) knots 0 0 0 0 0.062015 0.062015 0.12403 0.12403 0.172638 0.172638 0.221247 0.221247 0.221247 0.221247
  spline S173 degree 5 poles (715.665, -104.3709) (715.692, -104.3781) (715.8076, -104.4092) (716.012, -104.4635) (716.3057, -104.5401) (716.6891, -104.6373) (717.1357, -104.747) (717.5834, -104.8533) (718.0323, -104.9563) (718.4824, -105.056) (718.9335, -105.1524) (719.3858, -105.2457) (719.839, -105.336) (720.2932, -105.4234) (720.7483, -105.508) (721.2043, -105.5899) (721.661, -105.6691) (722.1187, -105.7457) (722.5771, -105.8197) (723.0363, -105.891) (723.4962, -105.9599) (723.957, -106.0262) (724.4184, -106.09) (724.8806, -106.1515) (725.3434, -106.2106) (725.8068, -106.2673) (726.271, -106.3218) (726.7357, -106.374) (727.2011, -106.4239) (727.667, -106.4716) (728.1336, -106.517) (728.6007, -106.5603) (729.0684, -106.6015) (729.5367, -106.6405) (730.0054, -106.6774) (730.4747, -106.7122) (730.9445, -106.745) (731.4148, -106.7757) (731.8856, -106.8043) (732.3569, -106.831) (732.8287, -106.8557) (733.3009, -106.8783) (733.7735, -106.8991) (734.2466, -106.9178) (734.7201, -106.9347) (735.1941, -106.9496) (735.6684, -106.9627) (736.1432, -106.9738) (736.6183, -106.9831) (737.0939, -106.9905) (737.5698, -106.9961) (738.0461, -106.9998) (738.5227, -107.0017) (738.9998, -107.0018) (739.4771, -107.0001) (739.9548, -106.9966) (740.4329, -106.9913) (740.9113, -106.9843) (741.39, -106.9755) (741.869, -106.965) (742.3483, -106.9527) (742.8279, -106.9387) (743.2118, -106.9262) (743.4999, -106.916) (743.692, -106.9088) (743.7881, -106.9052) knots 0.13851185 0.13851185 0.13851185 0.13851185 0.13851185 0.13851185 0.14285714 0.15714286 0.17142857 0.18571429 0.2 0.21428571 0.22857143 0.24285714 0.25714286 0.27142857 0.28571429 0.3 0.31428571 0.32857143 0.34285714 0.35714286 0.37142857 0.38571429 0.4 0.41428571 0.42857143 0.44285714 0.45714286 0.47142857 0.48571429 0.5 0.51428571 0.52857143 0.54285714 0.55714286 0.57142857 0.58571429 0.6 0.61428571 0.62857143 0.64285714 0.65714286 0.67142857 0.68571429 0.7 0.71428571 0.72857143 0.74285714 0.75714286 0.77142857 0.78571429 0.8 0.81428571 0.82857143 0.84285714 0.85714286 0.87142857 0.88571429 0.9 0.91428571 0.92857143 0.94285714 0.95714286 0.97142857 0.98571429 1 1 1 1 1 1
  arc A87 (743.7881, -106.9052) -> (747.5444, -97.8366) centre (452.3696, 19.1166) ccw
  spline S174 degree 5 poles (747.5444, -97.8366) (747.4791, -97.7661) (747.3483, -97.6252) (747.1518, -97.4143) (746.8892, -97.1339) (746.5599, -96.7849) (746.2297, -96.4373) (745.8984, -96.0911) (745.5661, -95.7464) (745.2329, -95.4032) (744.8986, -95.0614) (744.5632, -94.7212) (744.2269, -94.3824) (743.8895, -94.0452) (743.5511, -93.7095) (743.2117, -93.3753) (742.8712, -93.0427) (742.5297, -92.7117) (742.1872, -92.3823) (741.8436, -92.0545) (741.499, -91.7283) (741.1533, -91.4037) (740.8065, -91.0808) (740.4587, -90.7595) (740.1098, -90.44) (739.7599, -90.1221) (739.4089, -89.806) (739.0568, -89.4916) (738.7036, -89.179) (738.3494, -88.8681) (737.994, -88.5591) (737.6375, -88.2519) (737.28, -87.9465) (736.9213, -87.643) (736.5615, -87.3413) (736.2006, -87.0417) (735.8385, -86.7439) (735.4753, -86.4481) (735.1109, -86.1544) (734.7454, -85.8626) (734.3787, -85.573) (734.0109, -85.2854) (733.6418, -84.9999) (733.2716, -84.7166) (732.9002, -84.4354) (732.5275, -84.1565) (732.1536, -83.8799) (731.7784, -83.6057) (731.402, -83.3339) (731.0242, -83.0644) (730.6452, -82.7974) (730.2649, -82.5329) (729.8833, -82.271) (729.5003, -82.0116) (729.116, -81.755) (728.7302, -81.5011) (728.343, -81.2503) (727.9543, -81.0025) (727.564, -80.758) (727.1723, -80.5166) (726.7789, -80.2783) (726.4391, -80.076) (726.1773, -79.9225) (725.9943, -79.8163) (725.8906, -79.7565) (725.8664, -79.7426) knots -1 -1 -1 -1 -1 -1 -0.98571429 -0.97142857 -0.95714286 -0.94285714 -0.92857143 -0.91428571 -0.9 -0.88571429 -0.87142857 -0.85714286 -0.84285714 -0.82857143 -0.81428571 -0.8 -0.78571429 -0.77142857 -0.75714286 -0.74285714 -0.72857143 -0.71428571 -0.7 -0.68571429 -0.67142857 -0.65714286 -0.64285714 -0.62857143 -0.61428571 -0.6 -0.58571429 -0.57142857 -0.55714286 -0.54285714 -0.52857143 -0.51428571 -0.5 -0.48571429 -0.47142857 -0.45714286 -0.44285714 -0.42857143 -0.41428571 -0.4 -0.38571429 -0.37142857 -0.35714286 -0.34285714 -0.32857143 -0.31428571 -0.3 -0.28571429 -0.27142857 -0.25714286 -0.24285714 -0.22857143 -0.21428571 -0.2 -0.18571429 -0.17142857 -0.15714286 -0.14285714 -0.13851185 -0.13851185 -0.13851185 -0.13851185 -0.13851185 -0.13851185
  spline S175 degree 3 poles (725.1624, -77.8351) (725.0932, -78.0299) (725.0627, -78.2363) (725.0825, -78.6493) (725.1326, -78.8518) (725.2888, -79.1859) (725.3795, -79.3213) (725.5987, -79.5599) (725.726, -79.6618) (725.8664, -79.7426) knots 0 0 0 0 0.062015 0.062015 0.12403 0.12403 0.172638 0.172638 0.221247 0.221247 0.221247 0.221247
  arc A88 (725.1624, -77.8351) -> (727.8111, -70.0323) centre (452.3696, 19.1166) ccw
  spline S176 degree 3 poles (729.5308, -68.9475) (729.3259, -68.9202) (729.1177, -68.9332) (728.7178, -69.0384) (728.5301, -69.1295) (728.2358, -69.3517) (728.1221, -69.4685) (727.9342, -69.7325) (727.861, -69.8781) (727.8111, -70.0323) knots 0 0 0 0 0.062015 0.062015 0.12403 0.12403 0.172638 0.172638 0.221247 0.221247 0.221247 0.221247
  spline S177 degree 5 poles (729.5308, -68.9475) (729.5585, -68.9512) (729.6772, -68.9669) (729.887, -68.994) (730.1881, -69.0316) (730.581, -69.078) (731.038, -69.1284) (731.4958, -69.1754) (731.9543, -69.2189) (732.4135, -69.259) (732.8734, -69.2957) (733.334, -69.3292) (733.7951, -69.3595) (734.2568, -69.3869) (734.7191, -69.4114) (735.1818, -69.4331) (735.645, -69.452) (736.1087, -69.4682) (736.5729, -69.4817) (737.0375, -69.4925) (737.5025, -69.5007) (737.9679, -69.5063) (738.4337, -69.5094) (738.9, -69.51) (739.3665, -69.5082) (739.8334, -69.5039) (740.3007, -69.4973) (740.7683, -69.4884) (741.2362, -69.4772) (741.7044, -69.4636) (742.1729, -69.4478) (742.6417, -69.4298) (743.1107, -69.4095) (743.5801, -69.3871) (744.0496, -69.3625) (744.5195, -69.3357) (744.9895, -69.3069) (745.4598, -69.2759) (745.9303, -69.2429) (746.401, -69.2078) (746.872, -69.1707) (747.3431, -69.1315) (747.8144, -69.0904) (748.2859, -69.0473) (748.7576, -69.0022) (749.2294, -68.9551) (749.7014, -68.9061) (750.1735, -68.8552) (750.6458, -68.8024) (751.1183, -68.7477) (751.5909, -68.6911) (752.0636, -68.6326) (752.5364, -68.5723) (753.0094, -68.5101) (753.4824, -68.4461) (753.9556, -68.3803) (754.4289, -68.3127) (754.9022, -68.2432) (755.3757, -68.1721) (755.8492, -68.0991) (756.3228, -68.0244) (756.7965, -67.9479) (757.1755, -67.8853) (757.4598, -67.8376) (757.6493, -67.8054) (757.7441, -67.7893) knots 0.13851185 0.13851185 0.13851185 0.13851185 0.13851185 0.13851185 0.14285714 0.15714286 0.17142857 0.18571429 0.2 0.21428571 0.22857143 0.24285714 0.25714286 0.27142857 0.28571429 0.3 0.31428571 0.32857143 0.34285714 0.35714286 0.37142857 0.38571429 0.4 0.41428571 0.42857143 0.44285714 0.45714286 0.47142857 0.48571429 0.5 0.51428571 0.52857143 0.54285714 0.55714286 0.57142857 0.58571429 0.6 0.61428571 0.62857143 0.64285714 0.65714286 0.67142857 0.68571429 0.7 0.71428571 0.72857143 0.74285714 0.75714286 0.77142857 0.78571429 0.8 0.81428571 0.82857143 0.84285714 0.85714286 0.87142857 0.88571429 0.9 0.91428571 0.92857143 0.94285714 0.95714286 0.97142857 0.98571429 1 1 1 1 1 1
  arc A89 (757.7441, -67.7893) -> (760.2846, -58.308) centre (452.3696, 19.1166) ccw
  spline S178 degree 5 poles (760.2846, -58.308) (760.2106, -58.2466) (760.0625, -58.124) (759.8402, -57.9405) (759.5433, -57.6968) (759.1713, -57.3938) (758.7985, -57.0922) (758.4249, -56.7923) (758.0504, -56.4939) (757.6752, -56.1971) (757.2992, -55.9019) (756.9223, -55.6083) (756.5446, -55.3164) (756.1661, -55.0261) (755.7868, -54.7374) (755.4066, -54.4504) (755.0257, -54.1651) (754.6439, -53.8815) (754.2613, -53.5996) (753.8778, -53.3194) (753.4936, -53.041) (753.1085, -52.7643) (752.7225, -52.4894) (752.3358, -52.2163) (751.9482, -51.9451) (751.5598, -51.6756) (751.1705, -51.408) (750.7804, -51.1422) (750.3894, -50.8784) (749.9976, -50.6164) (749.6049, -50.3564) (749.2114, -50.0984) (748.8171, -49.8423) (748.4218, -49.5882) (748.0257, -49.3361) (747.6288, -49.0861) (747.231, -48.8381) (746.8323, -48.5923) (746.4327, -48.3486) (746.0322, -48.1071) (745.6308, -47.8677) (745.2286, -47.6306) (744.8254, -47.3957) (744.4214, -47.1632) (744.0164, -46.9329) (743.6105, -46.7051) (743.2037, -46.4797) (742.796, -46.2567) (742.3873, -46.0363) (741.9776, -45.8185) (741.567, -45.6033) (741.1554, -45.3907) (740.7428, -45.1808) (740.3293, -44.9736) (739.9148, -44.7693) (739.4992, -44.568) (739.0825, -44.3699) (738.6648, -44.175) (738.246, -43.9834) (737.826, -43.7952) (737.405, -43.6104) (737.0416, -43.4541) (736.762, -43.3361) (736.5667, -43.2547) (736.4561, -43.209) (736.4303, -43.1983) knots -1 -1 -1 -1 -1 -1 -0.98571429 -0.97142857 -0.95714286 -0.94285714 -0.92857143 -0.91428571 -0.9 -0.88571429 -0.87142857 -0.85714286 -0.84285714 -0.82857143 -0.81428571 -0.8 -0.78571429 -0.77142857 -0.75714286 -0.74285714 -0.72857143 -0.71428571 -0.7 -0.68571429 -0.67142857 -0.65714286 -0.64285714 -0.62857143 -0.61428571 -0.6 -0.58571429 -0.57142857 -0.55714286 -0.54285714 -0.52857143 -0.51428571 -0.5 -0.48571429 -0.47142857 -0.45714286 -0.44285714 -0.42857143 -0.41428571 -0.4 -0.38571429 -0.37142857 -0.35714286 -0.34285714 -0.32857143 -0.31428571 -0.3 -0.28571429 -0.27142857 -0.25714286 -0.24285714 -0.22857143 -0.21428571 -0.2 -0.18571429 -0.17142857 -0.15714286 -0.14285714 -0.13851185 -0.13851185 -0.13851185 -0.13851185 -0.13851185 -0.13851185
  spline S179 degree 3 poles (735.4834, -41.399) (735.4402, -41.6012) (735.4369, -41.8098) (735.5104, -42.2167) (735.5866, -42.411) (735.785, -42.7218) (735.8926, -42.8442) (736.1411, -43.0522) (736.2805, -43.1365) (736.4303, -43.1983) knots 0 0 0 0 0.062015 0.062015 0.12403 0.12403 0.172638 0.172638 0.221247 0.221247 0.221247 0.221247
  arc A90 (735.4834, -41.399) -> (737.0909, -33.3172) centre (452.3696, 19.1166) ccw